# Autodesk Inventor part: 14_WAY_HEADER
Saved by Autodesk Inventor 2015 SP1 (Build 190203100, 203)
## iProperties
Created: 2015-06-25
Part Number: 14_WAY_HEADER
Material: Generic
Document SubType Name: Modeling
Designer: Patrick
Density: 1 g/cm^3
Appearance: HEADER2MM, 14_WAY_HEADER
Author: Patrick
Autodesk Inventor part; units mm, degrees
ref_plane "YZ Plane" through (0, 0, 0) normal (1, 0, 0) x (0, 1, 0)
ref_plane "XZ Plane" through (0, 0, 0) normal (0, 1, 0) x (-1, 0, 0)
ref_plane "XY Plane" through (0, 0, 0) normal (0, 0, 1) x (1, 0, 0)
sketch "HEADER2MM, 14_WAY_HEADER_148" plane through (0, 0, 0) normal (0, 0, 1) x (1, 0, 0)
  line L0 (-3.3, -8.6) -> (-3.3, 8.6)
  line L1 (-3.3, 8.6) -> (3.3, 8.6)
  line L2 (3.3, 8.6) -> (3.3, -8.6)
  line L3 (3.3, -8.6) -> (-3.3, -8.6)
  constraints: 8 end point
extrude "Extrusion1" add sketch "HEADER2MM, 14_WAY_HEADER_148" along normal blind 1
body "Solid1"
